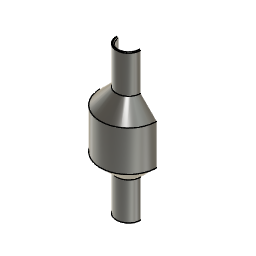
check valve 2 v2 (Autodesk Fusion 360 design; units mm, degrees)
Autodesk Fusion 360 part; units mm, degrees
note: some values were not read from the file. Set by a fixed rule: which sketch regions a step uses.
sketch "Skizze1" plane through (0, 0, 0) normal (1, 0, 0) x (0, 1, 0)
  line L0 (0, 65) -> (0, -75) construction
  line L1 (-6, 6) -> (-14, -2)
  line L2 (-14, -2) -> (-14, -12)
  line L3 (-21, -12) -> (15, -12) construction
  line L4 (-6, -30) -> (-14, -22)
  line L5 (-14, -22) -> (-14, -12)
  line L6 (-12.5, -2.6213) -> (-12.5, -12)
  line L7 (-3.7373, 6.1414) -> (-12.5, -2.6213)
  line L8 (-12.5, -21.3787) -> (-12.5, -12)
  line L9 (-3.7373, -30.1414) -> (-12.5, -21.3787)
  line L10 (-6, 24.5) -> (-6, 6)
  line L11 (-5, 24.2504) -> (-5, 11)
  line L12 (-3.6, 10.5) -> (-3.6, 6.2787)
  line L13 (-3.7373, 6.1414) -> (-3.6, 6.2787)
  line L14 (-4.1, 11) -> (-5, 11)
  line L15 (-5.7504, 24.75) -> (-5.5009, 24.7504)
  arc A0 (-5.7504, 24.75) -> (-6, 24.5) centre (-5.75, 24.5) ccw
  arc A1 (-5, 24.2504) -> (-5.5009, 24.7504) centre (-5.5, 24.2504) ccw
  arc A2 (-3.6, 10.5) -> (-4.1, 11) centre (-4.1, 10.5) ccw
  line L16 (-5, 15.9917) -> (-4.9, 12.9983)
  line L17 (-4.9, 12.9983) -> (-4.9, 11)
  line L18 (-6, -48.5) -> (-6, -30)
  arc A3 (-6, -48.5) -> (-5.7504, -48.75) centre (-5.75, -48.5) ccw
  line L19 (-5.7504, -48.75) -> (-5.5009, -48.7504)
  arc A4 (-5.5009, -48.7504) -> (-5, -48.2504) centre (-5.5, -48.2504) ccw
  line L20 (-5, -48.2504) -> (-5, -35)
  line L21 (-5, -39.9917) -> (-4.9, -36.9983)
  line L22 (-4.9, -36.9983) -> (-4.9, -35)
  line L23 (-4.1, -35) -> (-5, -35)
  arc A5 (-4.1, -35) -> (-3.6, -34.5) centre (-4.1, -34.5) ccw
  line L24 (-3.6, -34.5) -> (-3.6, -30.2787)
  line L25 (-3.7373, -30.1414) -> (-3.6, -30.2787)
  dimension "d6" = 14
  dimension "d7" = 10
  dimension "d64" = 6
  dimension "d65" = 5
  dimension "d67" = 3.6
  dimension "d68" = 0.25
  dimension "d69" = 0.5
  dimension "d70" = 0.5
  dimension "d71" = 0.1
  constraint vertical L0
  constraint vertical L2
  constraint perpendicular L0 L3
  constraint symmetric L1.start L3 L4.start
  constraint symmetric L1.end L3 L4.end
  constraint symmetric L2.end L3 L5.end
  constraint parallel L2 L6
  constraint parallel L1 L7
  constraint parallel L5 L8
  constraint parallel L4 L9
  constraint vertical L10
  constraint vertical L11
  constraint parallel L10 L12
  constraint parallel L7 L13
  constraint tangent L10 A0
  constraint tangent L15 A0
  constraint tangent L11 A1
  constraint tangent L15 A1
  constraint tangent L12 A2
  constraint tangent L14 A2
  constraint coincident L11 L16.start
  constraint coincident L14 L17.end
  constraint perpendicular L14 L17
  constraint symmetric L3 L11.end L20.end
  constraint symmetric L3 L12.end L24.end
  constraint symmetric L3 L10.start L18.start
  constraint symmetric L3 L15.start A3.end
  constraint symmetric L3 A0 A3
  constraint symmetric L3 L11.start A4.end
  constraint symmetric L3 L15.end L19.end
  constraint symmetric L3 A1 A4
  constraint symmetric L3 L12.start A5.end
  constraint symmetric L3 L14.start L23.start
  constraint symmetric L3 A2 A5
  constraint symmetric L3 L16.start L21.start
  constraint symmetric L3 L16.end L21.end
  constraint symmetric L3 L17.end L22.end
  constraint parallel L9 L25
  measures "d6" distance of L0 L2
  measures "d7" distance of L1.end L2.end
  measures "d64" distance of L0 L10
  measures "d65" distance of L0 L11
  measures "d67" distance of L0 L12
  measures "d68" radius of A0
  measures "d69" radius of A1
  measures "d70" radius of A2
  measures "d71" distance of L11 L17
revolve "Drehen1" add sketch "Skizze1" angle 360 about axis through (0, 0, 65) along (0, 0, -1) contours L1 L2 L4 L5 L6 L7 L8 L9 L10 L11 L12 L13 L14 L15 A0 A1 A2 L18 A3 L19 A4 L20 L23 A5 L24 L25 makes body 1
sketch "Skizze2" plane through (0, 0, 0) normal (1, 0, 0) x (0, 1, 0)
  circle A0 centre (-3.7, 23) radius 0.5
  line L0 (-3.7, 24) -> (-3.7, 10)
  circle A1 centre (-3.7, 19) radius 0.5
  line L1 (2.2, 25) -> (-2.2, 25)
  circle A2 centre (-3.7, 15) radius 0.5
  line L2 (-21, -12) -> (15, -12)
  circle A3 centre (-3.7, -47) radius 0.5
  circle A4 centre (-3.7, -43) radius 0.5
  circle A5 centre (-3.7, -39) radius 0.5
  dimension "d11" = 1
  dimension "d12" = 1
  dimension "d13" = 4
  dimension "d14" = 2
  dimension "d15" = 1
  dimension "d16" = 4
  constraint coincident A0.centre L0
  constraint coincident L0 A1.centre
  constraint coincident L0 A2.centre
  constraint symmetric A0 L2 A3
  constraint symmetric A1 L2 A4
  constraint symmetric A2 L2 A5
  measures "d11" diameter of A0
  measures "d12" diameter of A1
  measures "d13" distance of A0.centre A1.centre
  measures "d14" distance of A0.centre L1
  measures "d15" diameter of A2
  measures "d16" distance of A1.centre A2.centre
ref_plane "Arbeitsebene1" through (0, 0, -12) normal (0, 0, 1) x (1, 0, 0)
sketch "Skizze4" plane through (0, 0, -12) normal (0, 0, 1) x (1, 0, 0)
  line L0 (1, -12.5) -> (-1, -12.5)
  line L1 (-1, -12.5) -> (-1, -11)
  line L2 (-0.5, -10.5) -> (0.5, -10.5)
  line L3 (1, -11) -> (1, -12.5)
  line L4 (0, -6) -> (0, -14)
  arc A0 (-0.5, -10.5) -> (-1, -11) centre (-0.5, -11) ccw
  arc A1 (1, -11) -> (0.5, -10.5) centre (0.5, -11) ccw
  line L5 (-0.5, -10) -> (0.5, -10)
  arc A2 (1.5, -11) -> (0.5, -10) centre (0.5, -11) ccw
  line L6 (1.5, -11) -> (1.5, -13)
  line L7 (1.5, -13) -> (-1.5, -13)
  line L8 (-1.5, -13) -> (-1.5, -11)
  arc A3 (-0.5, -10) -> (-1.5, -11) centre (-0.5, -11) ccw
  dimension "d28" = 2
  dimension "d29" = 2
  dimension "d30" = 0.5
  dimension "d43" = 0.5
  constraint horizontal L0
  constraint vertical L1
  constraint horizontal L2
  constraint vertical L3
  constraint tangent L1 A0
  constraint tangent L2 A0
  constraint tangent L2 A1
  constraint tangent L3 A1
  constraint equal A0 A1
  measures "d28" distance of L1 L3
  measures "d29" distance of L0 L2
  measures "d30" radius of A0
extrude "Extrusion2" add sketch "Skizze4" along normal blind 11.4 separate body contours L0 L2 L3 L4 A1 | L0 L1 L2 L4 A0 makes body 2
extrude "Extrusion3" add sketch "Skizze4" against normal blind 11.4 separate body contours L0 L2 L3 L4 A1 | L0 L1 L2 L4 A0 makes body 3
mirror "Spiegeln1" about plane through (0, 0, 0) normal (0, 1, 0) of "Extrusion2" makes body 4
mirror "Spiegeln2" about plane through (0, 0, 0) normal (0, 1, 0) of "Extrusion3" makes body 5
sketch "Skizze5" plane through (0, 0, 0) normal (1, 0, 0) x (0, 1, 0)
  line L0 (0, 65) -> (0, -75)
  line L1 (-12.5, -2.6213) -> (0, 9.8787)
  line L2 (-12.5, -2.6213) -> (-12.5, -17.6213)
  line L3 (-12.5, -17.6213) -> (0, -17.6213)
  line L4 (-12, -2.8284) -> (0, 9.1716)
  line L5 (-12, -2.8284) -> (-12, -17.1213)
  line L6 (-12, -17.1213) -> (0, -17.1213)
  line L7 (0, -17.1213) -> (0, 9.8787)
  point P0 (-12.5, -2.6213)
  dimension "d39" = 17.6777
  dimension "d40" = 15
  constraint coincident P0 L1.start
  constraint coincident L0 L1.end
  constraint coincident L0 L3.end
  constraint perpendicular L0 L3
  constraint parallel L1 L4
  constraint parallel L2 L5
  constraint parallel L3 L6
  constraint coincident L0 L4.end
  measures "d39" distance of P0 L1.end
  measures "d40" distance of P0 L2.end
revolve "Drehen4" add sketch "Skizze5" angle 360 about axis through (0, 0, -17.1213) along (0, 0, 1) separate body contours L0 L4 L5 L6 L7 makes body 6
extrude "Extrusion4" cut sketch "Skizze4" along normal blind 13 bodies 6
extrude "Extrusion5" cut sketch "Skizze4" against normal blind 6.5 bodies 6
mirror "Spiegeln3" about plane through (0, 0, 0) normal (0, 1, 0) of "Extrusion5"
extrude "Extrusion6" cut 1 faces at (0.1667, 11.3264, -12) along direction (0, 0, 1) blind 14 on bodies 6 bodies 6
sketch "Skizze6" plane through (0, 0, 0) normal (1, 0, 0) x (0, 1, 0)
  spline S0 degree 5 poles (-8.6987, -17.149) (-8.4951, -16.7769) (-8.0722, -16.0652) (-7.3908, -15.095) (-6.3797, -13.9824) (-4.8475, -12.8859) (-3.2632, -12.2903) (-1.7696, -12.0528) (-0.6162, -12) (0, -12) knots 0 0 0 0 0 0 0.2 0.4 0.6 0.8 1 1 1 1 1 1
  line L0 (-1.5, -12) -> (1.5, -12)
  line L1 (-9.1943, -18.0546) -> (-8.2031, -16.2434)
  line L2 (0, 65) -> (0, -75)
  line L3 (0, -12) -> (0, -17.149)
  line L4 (-8.6987, -17.149) -> (0, -17.149)
  point P0 (0, -12)
  constraint coincident P0 S0.end
  constraint midpoint P0 L0
  constraint midpoint S0.start L1
  constraint coincident L2 L3.end
  constraint parallel L2 L3
  constraint perpendicular L3 L4
revolve "Drehen5" cut sketch "Skizze6" angle 360 about axis through (0, 0, 65) along (0, 0, -1) bodies 6
sketch "Skizze7" plane through (0, 0, -17.1213) normal (0, 0, -1) x (1, 0, 0)
  spline S0 degree 3 poles (0, 8.6835) (0.9903, 8.6835) (1.9745, 8.5141) (3.9749, 7.8027) (4.956, 7.2194) (6.6396, 5.7095) (7.3258, 4.7973) (8.3101, 2.7613) (8.5986, 1.6569) (8.7362, -0.6004) (8.5839, -1.7316) (7.8542, -3.8721) (7.2838, -4.8609) (5.7961, -6.5641) (4.893, -7.2622) (2.8701, -8.2731) (1.7696, -8.5762) (-0.4857, -8.7433) (-1.6188, -8.6059) (-3.7687, -7.9043) (-4.7649, -7.347) (-6.4874, -5.8818) (-7.1974, -4.9879) (-8.2347, -2.9784) (-8.5522, -1.882) (-8.749, 0.3709) (-8.6264, 1.5058) (-7.9531, 3.6647) (-7.4089, 4.668) (-6.2793, 6.0319) (-5.8176, 6.4783) (-4.8046, 7.2615) (-4.2564, 7.5958) (-3.6764, 7.8669) (-2.652, 8.3456) (-1.5439, 8.6196) (-0.2763, 8.6802) (-0.1381, 8.6835) (0, 8.6835) knots 0.380725 0.380725 0.380725 0.380725 0.678433 0.678433 1.01765 1.01765 1.356866 1.356866 1.696083 1.696083 2.035299 2.035299 2.374516 2.374516 2.713732 2.713732 3.052949 3.052949 3.392165 3.392165 3.731382 3.731382 4.070598 4.070598 4.409815 4.409815 4.749031 4.749031 5.088248 5.088248 5.280309 5.280309 5.472371 5.472371 5.472371 5.811587 5.811587 5.853096 5.853096 5.853096 5.853096
  line L0 (-1.5, -11.9059) -> (-1.5, -11)
  arc A0 (-0.5, -10) -> (-1.5, -11) centre (-0.5, -11) ccw
  line L1 (-0.5, -10) -> (0.5, -10)
  arc A1 (1.5, -11) -> (0.5, -10) centre (0.5, -11) ccw
  line L2 (1.5, -11) -> (1.5, -11.9059)
  arc A2 (1.5, -11.9059) -> (1.5, 11.9059) centre (0, 0) ccw
  line L3 (1.5, 11.9059) -> (1.5, 11)
  arc A3 (0.5, 10) -> (1.5, 11) centre (0.5, 11) ccw
  line L4 (0.5, 10) -> (-0.5, 10)
  arc A4 (-1.5, 11) -> (-0.5, 10) centre (-0.5, 11) ccw
  line L5 (-1.5, 11) -> (-1.5, 11.9059)
  arc A5 (-1.5, 11.9059) -> (-1.5, -11.9059) centre (0, 0) ccw
  spline S1 degree 5 poles (1.5, 11.9059) (1.8388, 11.7751) (2.5001, 11.5019) (3.4429, 11.0566) (4.6015, 10.392) (5.8829, 9.4422) (6.9947, 8.3736) (7.9337, 7.1895) (8.6984, 5.8976) (9.2892, 4.5118) (9.7084, 3.0512) (9.9585, 1.5389) (10.0415, 0) (9.9585, -1.5389) (9.7084, -3.0512) (9.2892, -4.5118) (8.6984, -5.8976) (7.9337, -7.1895) (6.9947, -8.3736) (5.8829, -9.4422) (4.6015, -10.392) (3.4429, -11.0566) (2.5001, -11.5019) (1.8388, -11.7751) (1.5, -11.9059) knots 0 0 0 0 0 0 0.05 0.1 0.15 0.2 0.25 0.3 0.35 0.4 0.45 0.5 0.55 0.6 0.65 0.7 0.75 0.8 0.85 0.9 0.95 1 1 1 1 1 1
  line L6 (0, 6) -> (0, 14)
  spline S2 degree 5 poles (-1.5, 11.9059) (-1.8388, 11.7751) (-2.5001, 11.5019) (-3.4429, 11.0566) (-4.6015, 10.392) (-5.8829, 9.4422) (-6.9947, 8.3736) (-7.9337, 7.1895) (-8.6984, 5.8976) (-9.2892, 4.5118) (-9.7084, 3.0512) (-9.9585, 1.5389) (-10.0415, 0) (-9.9585, -1.5389) (-9.7084, -3.0512) (-9.2892, -4.5118) (-8.6984, -5.8976) (-7.9337, -7.1895) (-6.9947, -8.3736) (-5.8829, -9.4422) (-4.6015, -10.392) (-3.4429, -11.0566) (-2.5001, -11.5019) (-1.8388, -11.7751) (-1.5, -11.9059) knots 0 0 0 0 0 0 0.05 0.1 0.15 0.2 0.25 0.3 0.35 0.4 0.45 0.5 0.55 0.6 0.65 0.7 0.75 0.8 0.85 0.9 0.95 1 1 1 1 1 1
  line L7 (-1.2006, 12.948) -> (4.2006, 10.8638)
  line L8 (4.2006, -10.8638) -> (-1.2006, -12.948)
  line L9 (1.2006, 12.948) -> (-4.2006, 10.8638)
  line L10 (-4.2006, -10.8638) -> (1.2006, -12.948)
  point P0 (8, 7)
  point P1 (10, 0)
  point P2 (8, -7)
  point P3 (-8, 7)
  point P4 (-10, 0)
  point P5 (-8, -7)
  constraint coincident A2.end L3.start
  constraint coincident L2.end A2.start
  constraint midpoint A2.end L7
  constraint midpoint L2.end L8
  constraint symmetric A2.end L6 L5.end
  constraint symmetric P0 L6 P3
  constraint symmetric P1 L6 P4
  constraint symmetric P2 L6 P5
  constraint symmetric L2.end L6 L0.start
  constraint symmetric L6 L7.start L9.start
  constraint symmetric L6 L7.end L9.end
  constraint symmetric L6 L8.start L10.start
  constraint symmetric L6 L8.end L10.end
extrude "Extrusion7" cut sketch "Skizze7" against normal blind 22 contours A5 S2 | A2 S1 bodies 6
sketch "Skizze8" plane through (0, 0, 0) normal (0, 1, 0) x (1, 0, 0)
  line L0 (10.2242, 11.8319) -> (6, 15)
  line L1 (6, 15) -> (6, 18)
  line L2 (6, 18) -> (10.2242, 18)
  line L3 (10.2242, 18) -> (10.2242, 11.8319)
  constraint vertical L1
  constraint perpendicular L1 L2
  constraint perpendicular L2 L3
revolve "Drehen6" cut sketch "Skizze8" angle 15 about axis through (0, 0, 65) along (0, 0, -1) second angle 15 bodies 6
mirror "Spiegeln4" about plane through (0, 0, 0) normal (1, 0, 0) of "Drehen6"
combine "Kombinieren1" operation add target body 4 tool bodies 5
combine "Kombinieren2" operation add target body 2 tool bodies 3
ref_plane "Arbeitsebene2" through (-14, 0, -12.7609) normal (-1, 0, 0) x (0, 1, 0)
sketch "Skizze9" plane through (-14, 0, -12.7609) normal (-1, 0, 0) x (0, 1, 0)
  line L0 (0.017, 2.534) -> (-2.483, 0.034)
  line L1 (-2.483, 0.034) -> (-0.983, 0.034)
  line L2 (-0.983, 0.034) -> (-0.983, -4.966)
  line L3 (-0.983, -4.966) -> (0.017, -4.966)
  line L4 (0.017, 2.534) -> (2.517, 0.034)
  line L5 (0.017, -4.966) -> (1.017, -4.966)
  line L6 (1.017, -4.966) -> (1.017, 0.034)
  line L7 (1.017, 0.034) -> (2.517, 0.034)
  constraint perpendicular L1 L2
  constraint perpendicular L2 L3
  constraint parallel L3 L5
  constraint perpendicular L5 L6
  constraint perpendicular L6 L7
extrude "Extrusion8" add sketch "Skizze9" against normal blind 0.5 bodies 1
extrude "Extrusion9" add 1 faces at (-14, 0.017, -11.1283) along direction (-1, 0, 0) blind 0.5 on bodies 1 bodies 1
combine "Kombinieren3" operation add target body 1 tool bodies 2 4
named bodies: "body", "guide1", "guide2", "bulb"
